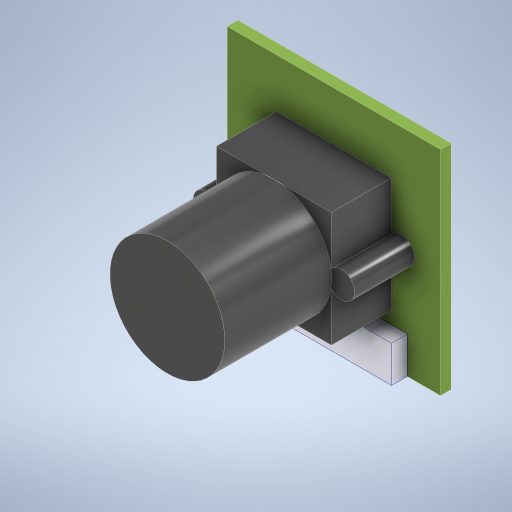
# Autodesk Inventor part: PiCam
Saved by Autodesk Inventor 2023 (Build 270158000, 158)
## iProperties
Created: 2022-07-24
Part Number: PiCam
Material: Genérico
Document SubType Name: Modeling
Designer: LJNC
Density: 1 g/cm^3
Appearance: Valor por defecto
Author: LJNC
Autodesk Inventor part; units mm, degrees
ref_plane "YZ Plane" through (0, 0, 0) normal (1, 0, 0) x (0, 1, 0)
ref_plane "XZ Plane" through (0, 0, 0) normal (0, 1, 0) x (-1, 0, 0)
ref_plane "XY Plane" through (0, 0, 0) normal (0, 0, 1) x (1, 0, 0)
sketch "Boceto1" plane through (0, 0, 0) normal (0, 0, 1) x (1, 0, 0)
  line L0 (-16, 16) -> (16, 16)
  line L1 (16, 16) -> (16, -16)
  line L2 (16, -16) -> (-16, -16)
  line L3 (-16, -16) -> (-16, 16)
  line L4 (-16, 0) -> (16, 0) construction
  line L5 (-11, -10.5) -> (11, -10.5)
  line L6 (11, -10.5) -> (11, -16)
  line L7 (11, -16) -> (-11, -16)
  line L8 (-11, -16) -> (-11, -10.5)
  line L9 (-8.625, 8.625) -> (8.625, 8.625)
  line L10 (8.625, 8.625) -> (8.625, -8.625)
  line L11 (8.625, -8.625) -> (-8.625, -8.625)
  line L12 (-8.625, -8.625) -> (-8.625, 8.625)
  line L13 (0, 0) -> (0, 8.625) construction
  circle A0 centre (10.125, 0) radius 2
  line L14 (0, 0) -> (10.125, 0) construction
  circle A1 centre (-10.125, 0) radius 2
  circle A2 centre (0, 0) radius 8.625
  circle A3 centre (-13.625, 14) radius 0.5
  point P0 (0, -16)
  point P1 (-8.625, 0)
  point P2 (-8.625, 1.3229)
  point P3 (-8.625, -1.3229)
  point P4 (8.625, -1.3229)
  point P5 (8.625, 1.3229)
  point P6 (-8.5386, 1.2179)
  point P7 (-8.5386, -1.2179)
  point P8 (8.5386, -1.2179)
  point P9 (8.5386, 1.2179)
  dimension "d0" = 32
  dimension "d1" = 22
  dimension "d2" = 5.5
  dimension "d3" = 17.25
  dimension "d4" = 4
  dimension "d6" = 1.5
  dimension "d7" = 1.5
  dimension "d16" = 13.625
  dimension "d17" = 2
  dimension "d18" = 1
  constraints: 30 end point, 7 midpoint, 6 parallel, 5 perpendicular, 4 centre point, 4 horizontal, 2 coincident, 2 point on line, 1 equal radius, 1 tangent, 1 vertical
  measures "d0" distance of L0.start L0.end
  measures "d1" distance of L6.end L7.end
  measures "d2" distance of L7.end L5.start
  measures "d3" distance of L9.start L9.end
  measures "d4" diameter of A0
  measures "d6" distance from line of L10 L14.end
  measures "d7" distance from line of L12 A1.centre
  measures "d16" horizontal distance of L13.end A3.centre
  measures "d17" distance from line of L0 A3.centre
  measures "d18" diameter of A3
extrude "Extrusión1" add sketch "Boceto1" along normal blind 9 contours L9 A2 A1 L12 | L9 L10 A0 A2 | A2 A0 A1 | A1 A2 L12 | L12 A1 | A2 A0 | A0 L10 A2 | A1 A2 | A2 A1 L12 | A1 A2 L11 L12 | A0 L10 | A2 L10 A0 | A0 L10 L11 A2
extrude "Extrusión2" add sketch "Boceto1" against normal blind 1.61 separate body contours L0 L1 L2 L6 L5 L8 L3 | L8 L5 L6 L2 | L9 A2 A1 L12 | L9 L10 A0 A2 | A2 A0 A1 | A1 A2 L12 | L12 A1 | A2 A0 | A0 L10 A2 | A1 A2 | A2 A1 L12 | A1 A2 L11 L12 | A0 L10 | A2 L10 A0 | A0 L10 L11 A2 | A3
extrude "Extrusión3" add sketch "Boceto1" along normal blind 2.35 separate body contours L8 L5 L6 L2
extrude "Extrusión4" add sketch "Boceto1" along normal blind 25 contours A2 A0 A1 | A2 A0 | A1 A2 bodies 1
equation "\"d7\" = d6"
